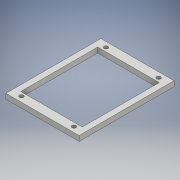
# Autodesk Inventor part: Uzupelnienie_podwozia
Saved by Autodesk Inventor 2018 (Build 220112000, 112)
## iProperties
Created: 2019-10-16
Part Number: Uzupelnienie_podwozia
Material: Ogólny
Document SubType Name: Modeling
Designer: Raven
Density: 1 g/cm^3
Appearance: Domyślna
Author: Raven
Autodesk Inventor part; units mm, degrees
ref_plane "YZ Plane" through (0, 0, 0) normal (1, 0, 0) x (0, 1, 0)
ref_plane "XZ Plane" through (0, 0, 0) normal (0, 1, 0) x (-1, 0, 0)
ref_plane "XY Plane" through (0, 0, 0) normal (0, 0, 1) x (1, 0, 0)
sketch "Szkic1" plane through (0, 0, 0) normal (0, 0, 1) x (1, 0, 0)
  line L0 (0, 0) -> (57, 0)
  line L1 (57, 0) -> (57, 74)
  line L2 (57, 74) -> (0, 74)
  line L3 (0, 74) -> (0, 0)
  line L4 (28.5, 74) -> (28.5, 67) construction
  line L5 (0, 37) -> (4.5, 37) construction
  line L6 (28.5, 0) -> (28.5, 7) construction
  line L7 (57, 37) -> (52.5, 37) construction
  line L8 (4.5, 7) -> (52.5, 7)
  line L9 (52.5, 7) -> (52.5, 67)
  line L10 (52.5, 67) -> (4.5, 67)
  line L11 (4.5, 67) -> (4.5, 7)
  line L12 (57, 0) -> (49, 0) construction
  line L13 (0, 0) -> (8, 0) construction
  line L14 (8, 0) -> (8, 4) construction
  line L15 (49, 0) -> (49, 4) construction
  circle A0 centre (49, 4) radius 1.55
  circle A1 centre (8, 4) radius 1.55
  line L16 (57, 74) -> (49, 74) construction
  line L17 (49, 74) -> (49, 70) construction
  line L18 (0, 74) -> (8, 74) construction
  line L19 (8, 74) -> (8, 70) construction
  circle A2 centre (8, 70) radius 1.55
  circle A3 centre (49, 70) radius 1.55
  dimension "d0" = 57
  dimension "d1" = 74
  dimension "d2" = 7
  dimension "d3" = 4.5
  dimension "d4" = 7
  dimension "d5" = 4.5
  dimension "d6" = 8
  dimension "d7" = 8
  dimension "d8" = 4
  dimension "d9" = 3.1
  dimension "d10" = 3.1
  dimension "d11" = 4
  dimension "d12" = 3.1
  dimension "d13" = 3.1
  constraints: 40 end point, 4 centre point, 4 coincident, 4 horizontal, 4 midpoint, 4 parallel, 4 perpendicular, 4 point on line, 4 vertical
  measures "d0" distance of L2.end L1.end
  measures "d1" distance of L1.end L0.end
  measures "d2" distance of L4.start L4.end
  measures "d3" distance of L5.start L5.end
  measures "d4" distance of L6.start L6.end
  measures "d5" distance of L7.start L7.end
  measures "d6" distance of L0.end L12.end
  measures "d7" distance of L0.start L13.end
  measures "d8" distance of L13.end L14.end
  measures "d9" diameter of A0
  measures "d10" diameter of A1
  measures "d11" distance of L16.end L17.end
  measures "d12" diameter of A2
  measures "d13" diameter of A3
extrude "Wyciągnięcie proste1" add sketch "Szkic1" along normal blind 4
